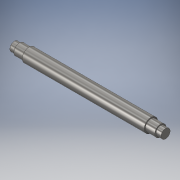
# Autodesk Inventor part: Stopper Axle
Saved by Autodesk Inventor 2019.4 (Build 234330000, 330)
## iProperties
Created: 2019-10-20
Part Number: Stopper Axle
Material: Stainless Steel
Document SubType Name: Modeling
Designer: admin
Density: 8 g/cm^3
Appearance: Semi-Polished
Author: admin
Autodesk Inventor part; units mm, degrees
ref_plane "YZ Plane" through (0, 0, 0) normal (1, 0, 0) x (0, 1, 0)
ref_plane "XZ Plane" through (0, 0, 0) normal (0, 1, 0) x (-1, 0, 0)
ref_plane "XY Plane" through (0, 0, 0) normal (0, 0, 1) x (1, 0, 0)
sketch "Sketch1" plane through (0, 0, 0) normal (0, 0, 1) x (1, 0, 0)
  line L0 (0, 0) -> (0, 4)
  line L1 (0, 4) -> (4.5, 4)
  line L2 (4.5, 4) -> (4.5, 5)
  line L3 (4.5, 5) -> (12.9, 5)
  line L4 (12.9, 5) -> (12.9, 6)
  line L5 (12.9, 6) -> (120.5, 6)
  line L6 (120.5, 6) -> (120.5, 5)
  line L7 (120.5, 5) -> (128.9, 5)
  line L8 (128.9, 5) -> (128.9, 4)
  line L9 (128.9, 4) -> (133.4, 4)
  line L10 (133.4, 4) -> (133.4, 0)
  line L11 (133.4, 0) -> (0, 0)
  line L12 (66.7, 6) -> (66.7, 0) construction
  dimension "d0" = 4
  dimension "d1" = 5
  dimension "d2" = 6
  dimension "d3" = 4.5
  dimension "d4" = 107.6
  dimension "d5" = 124.4
  dimension "d6" = 4.5
  constraints: 26 end point, 9 perpendicular, 4 point on line, 2 midpoint, 1 horizontal, 1 vertical
  measures "d0" distance between parallel lines of L11 L1
  measures "d1" distance between parallel lines of L11 L3
  measures "d2" distance between parallel lines of L11 L5
  measures "d3" distance of L0.end L1.end
  measures "d4" distance of L4.end L5.end
  measures "d5" distance between parallel lines of L8 L2
  measures "d6" distance of L8.end L9.end
revolve "Revolution1" add sketch "Sketch1" angle 360 about axis through (133.4, 0, 0) along (-1, 0, 0)
body "Solid1"
